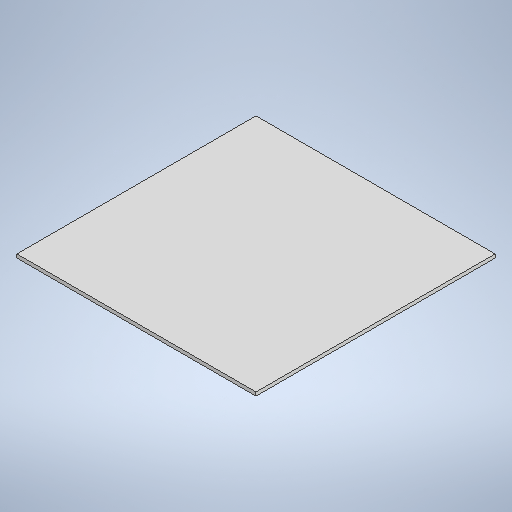
# Autodesk Inventor part: podstawa_plyta_200_200_3
Saved by Autodesk Inventor 2025.2 (Build 292293000, 293)
## iProperties
Created: 2025-03-19
Part Number: podstawa_plyta_200_200_3
Material: Ogólny
Document SubType Name: Modeling
Designer: tadek
Density: 1 g/cm^3
Appearance: Domyślna
Author: tadek
Autodesk Inventor part; units mm, degrees
ref_plane "YZ Plane" through (0, 0, 0) normal (1, 0, 0) x (0, 1, 0)
ref_plane "XZ Plane" through (0, 0, 0) normal (0, 1, 0) x (-1, 0, 0)
ref_plane "XY Plane" through (0, 0, 0) normal (0, 0, 1) x (1, 0, 0)
sketch "Szkic1" plane through (0, 0, 0) normal (0, 1, 0) x (-1, 0, 0)
  line L0 (0, 0) -> (1000, 0) construction
  line L1 (1000, 0) -> (1000, -1000)
  line L2 (1000, -1000) -> (0, -1000)
  line L3 (0, -1000) -> (0, 0) construction
  line L4 (1000, 0) -> (1000, 1000)
  line L5 (1000, 1000) -> (0, 1000)
  line L6 (-1000, 0) -> (-1000, -1000)
  line L7 (-1000, -1000) -> (0, -1000)
  line L8 (-1000, 0) -> (-1000, 1000)
  line L9 (-1000, 1000) -> (0, 1000)
  point P0 (500, -1000)
  point P1 (500, 0)
  dimension "d0" = 1000
  dimension "d1" = 1000
  constraints: 20 end point, 5 symmetric about line, 2 midpoint, 2 parallel, 1 horizontal, 1 perpendicular
  measures "d0" distance of L1.end L2.end
  measures "d1" distance of point (500, -1000) point (500, 0)
extrude "Wyciągnięcie proste1" add sketch "Szkic1" along normal blind 30
